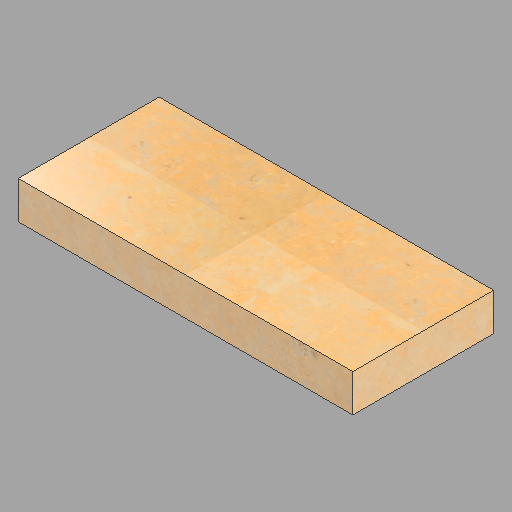
# Autodesk Inventor part: cap - 10
Saved by Autodesk Inventor 2023 (Build 270158030, 158C)
## iProperties
RuleStatus: InUse
Created: 2022-03-21
Part Number: cap - 10
Material: Granite, Cut, Polished
Document SubType Name: Modeling
Designer: awelt
Mass: 94573.8 g
Surface Area: 9508.05 cm^2
Volume: 35027.3 cm^3
Density: 2.7 g/cm^3
Appearance: Amber Select
AfterDocSave0: Convert in3 volume to ft3
in3 to ft3: 1.24
TEST: 1.237
Author: awelt
Autodesk Inventor part; units mm, degrees
ref_plane "YZ Plane" through (0, 0, 0) normal (1, 0, 0) x (0, 1, 0)
ref_plane "XZ Plane" through (0, 0, 0) normal (0, 1, 0) x (-1, 0, 0)
ref_plane "XY Plane" through (0, 0, 0) normal (0, 0, 1) x (1, 0, 0)
sketch "Sketch1" plane through (0, 0, 0) normal (0, 1, 0) x (-1, 0, 0)
  line L0 (452.4375, -190.5) -> (-452.4375, -190.5)
  line L1 (-452.4375, -190.5) -> (-452.4375, 190.5)
  line L2 (-452.4375, 190.5) -> (452.4375, 190.5)
  line L3 (452.4375, 190.5) -> (452.4375, -190.5)
  line L4 (452.4375, -190.5) -> (-452.4375, 190.5) construction
  line L5 (-452.4375, -190.5) -> (452.4375, 190.5) construction
  point P0 (0, 0)
  dimension "d0" = 904.875
  dimension "d1" = 381
  constraints: 12 end point, 2 midpoint, 2 parallel, 1 horizontal, 1 perpendicular
  measures "d0" distance of L1.end L2.end
  measures "d1" distance of L0.end L1.end
extrude "Extrusion1" add sketch "Sketch1" along normal blind 101.6
body "Solid1"
